barrel microswtich mount - front_v3 (Autodesk Fusion 360 design; units mm, degrees)
Autodesk Fusion 360 part; units mm, degrees
sketch "Sketch1" plane through (0, 0, 0) normal (0, 1, 0) x (1, 0, 0)
  line L0 (-4.4022, -9.8222) -> (-3.1214, -8.5414)
  arc A0 (10, -4.8314) -> (9.8222, -4.4022) centre (9.3929, -4.8314) ccw
  line L1 (6.5607, -5.5) -> (3.9, -2.8393)
  line L2 (-9.9987, -4.7917) -> (-10, -9.5)
  line L3 (9.8222, -4.4022) -> (8.5414, -3.1214)
  arc A1 (-3.2628, 8.2) -> (-3.1214, 8.5414) centre (-3.2628, 8.4) ccw
  line L4 (3.9, 2.8393) -> (6.5607, 5.5)
  arc A2 (-8.5414, 3.1214) -> (-8.2, 3.2628) centre (-8.4, 3.2628) ccw
  line L5 (-4.8314, 10) -> (-9.5, 10)
  line L6 (-6.5607, 5.5) -> (-3.9, 2.8393)
  arc A3 (-9.5, 10) -> (-10, 9.5) centre (-9.5, 9.5) ccw
  arc A4 (8.2, 3.2628) -> (8.5414, 3.1214) centre (8.4, 3.2628) ccw
  line L7 (-5.5, 6.5607) -> (-5.5, 8.2)
  line L8 (6.5607, 5.5) -> (8.2, 5.5)
  line L9 (8.5414, 3.1214) -> (9.8222, 4.4022)
  arc A5 (3.1214, 8.5414) -> (3.2628, 8.2) centre (3.2628, 8.4) ccw
  line L10 (-8.2, 3.2628) -> (-8.2, 5.5)
  line L11 (9.5, 10) -> (4.8314, 10)
  arc A6 (10, 9.5) -> (9.5, 10) centre (9.5, 9.5) ccw
  line L12 (10, 4.8314) -> (10, 9.5)
  arc A7 (-4.4312, 9.8494) -> (-4.8314, 10) centre (-4.8314, 9.3929) ccw
  line L13 (-9.8494, 4.4312) -> (-8.5414, 3.1214)
  line L14 (4.4022, 9.8222) -> (3.1214, 8.5414)
  line L15 (-5.5, 8.2) -> (-3.2628, 8.2)
  line L16 (5.5, 8.2) -> (5.5, 6.5607)
  arc A8 (-10, 4.9) -> (-9.8494, 4.4312) centre (-9.3734, 4.8428) ccw
  circle A9 centre (0, 0) radius 2.1
  arc A10 (4.8314, 10) -> (4.4022, 9.8222) centre (4.8314, 9.3929) ccw
  line L17 (-2.8393, 3.9) -> (-5.5, 6.5607)
  line L18 (5.5, 6.5607) -> (2.8393, 3.9)
  line L19 (-3.9, 2.8393) -> (-3.9, -2.8393)
  line L20 (-10, 9.5) -> (-10, 4.9)
  line L21 (2.8393, 3.9) -> (-2.8393, 3.9)
  line L22 (3.9, -2.8393) -> (3.9, 2.8393)
  line L23 (3.2628, 8.2) -> (5.5, 8.2)
  line L24 (8.2, 5.5) -> (8.2, 3.2628)
  line L25 (5.5, -6.5607) -> (5.5, -8.2)
  arc A11 (4.2336, -9.6536) -> (4.8314, -10) centre (4.8837, -9.2207) ccw
  arc A12 (-4.8314, -10) -> (-4.4022, -9.8222) centre (-4.8314, -9.3929) ccw
  line L26 (-5.5, -6.5607) -> (-2.8393, -3.9)
  line L27 (10, -9.5) -> (10, -4.8314)
  line L28 (-8.5414, -3.1214) -> (-9.8222, -4.4022)
  line L29 (5.5, -8.2) -> (3.2628, -8.2)
  line L30 (4.8314, -10) -> (9.5, -10)
  line L31 (-8.2, -5.5) -> (-8.2, -3.2628)
  arc A13 (8.5414, -3.1214) -> (8.2, -3.2628) centre (8.4, -3.2628) ccw
  line L32 (-2.8393, -3.9) -> (2.8393, -3.9)
  arc A14 (-8.2, -3.2628) -> (-8.5414, -3.1214) centre (-8.4, -3.2628) ccw
  arc A15 (-3.1214, -8.5414) -> (-3.2628, -8.2) centre (-3.2628, -8.4) ccw
  line L33 (3.1214, -8.5414) -> (4.2336, -9.6536)
  line L34 (-5.5, -8.2) -> (-5.5, -6.5607)
  line L35 (-6.5607, -5.5) -> (-8.2, -5.5)
  line L36 (8.2, -3.2628) -> (8.2, -5.5)
  arc A16 (-9.8222, -4.4022) -> (-9.9987, -4.7917) centre (-9.3929, -4.8314) ccw
  line L37 (-9.5, -10) -> (-4.8314, -10)
  arc A17 (-10, -9.5) -> (-9.5, -10) centre (-9.5, -9.5) ccw
  arc A18 (3.2628, -8.2) -> (3.1214, -8.5414) centre (3.2628, -8.4) ccw
  line L38 (8.2, -5.5) -> (6.5607, -5.5)
  line L39 (-3.2628, -8.2) -> (-5.5, -8.2)
  line L40 (-3.9, -2.8393) -> (-6.5607, -5.5)
  line L41 (2.8393, -3.9) -> (5.5, -6.5607)
  arc A19 (9.5, -10) -> (10, -9.5) centre (9.5, -9.5) ccw
  line L42 (-3.1214, 8.5414) -> (-4.4312, 9.8494)
  arc A20 (9.8222, 4.4022) -> (10, 4.8314) centre (9.3929, 4.8314) ccw
  line L43 (-8.2, 5.5) -> (-6.5607, 5.5)
  line L44 (4, 2.7979) -> (6.6021, 5.4)
  line L45 (6.6021, 5.4) -> (8.1, 5.4)
  line L46 (8.1, 5.4) -> (8.1, 3.2628)
  arc A21 (8.1, 3.2628) -> (8.6121, 3.0507) centre (8.4, 3.2628) ccw
  line L47 (8.6121, 3.0507) -> (9.8929, 4.3315)
  arc A22 (9.8929, 4.3315) -> (10.1, 4.8314) centre (9.3929, 4.8314) ccw
  line L48 (10.1, 4.8314) -> (10.1, 9.5)
  arc A23 (10.1, 9.5) -> (9.5, 10.1) centre (9.5, 9.5) ccw
  line L49 (9.5, 10.1) -> (4.8314, 10.1)
  arc A24 (4.8314, 10.1) -> (4.3315, 9.8929) centre (4.8314, 9.3929) ccw
  line L50 (4.3315, 9.8929) -> (3.0507, 8.6121)
  arc A25 (3.0507, 8.6121) -> (3.2628, 8.1) centre (3.2628, 8.4) ccw
  line L51 (3.2628, 8.1) -> (5.4, 8.1)
  line L52 (5.4, 8.1) -> (5.4, 6.6021)
  line L53 (5.4, 6.6021) -> (2.7979, 4)
  line L54 (2.7979, 4) -> (-2.7979, 4)
  line L55 (-2.7979, 4) -> (-5.4, 6.6021)
  line L56 (-5.4, 6.6021) -> (-5.4, 8.1)
  line L57 (-5.4, 8.1) -> (-3.2628, 8.1)
  arc A26 (-3.2628, 8.1) -> (-3.0509, 8.6124) centre (-3.2628, 8.4) ccw
  line L58 (-3.0509, 8.6124) -> (-4.3627, 9.9223)
  arc A27 (-4.3627, 9.9223) -> (-4.8314, 10.1) centre (-4.8314, 9.3929) ccw
  line L59 (-4.8314, 10.1) -> (-9.5, 10.1)
  arc A28 (-9.5, 10.1) -> (-10.1, 9.5) centre (-9.5, 9.5) ccw
  line L60 (-10.1, 9.5) -> (-10.1, 4.9044)
  arc A29 (-10.1, 4.9044) -> (-9.9226, 4.363) centre (-9.3734, 4.8428) ccw
  line L61 (-9.9226, 4.363) -> (-8.6124, 3.0509)
  arc A30 (-8.6124, 3.0509) -> (-8.1, 3.2628) centre (-8.4, 3.2628) ccw
  line L62 (-8.1, 3.2628) -> (-8.1, 5.4)
  line L63 (-8.1, 5.4) -> (-6.6021, 5.4)
  line L64 (-6.6021, 5.4) -> (-4, 2.7979)
  line L65 (-4, 2.7979) -> (-4, -2.7979)
  line L66 (-4, -2.7979) -> (-6.6021, -5.4)
  line L67 (-6.6021, -5.4) -> (-8.1, -5.4)
  line L68 (-8.1, -5.4) -> (-8.1, -3.2628)
  arc A31 (-8.1, -3.2628) -> (-8.6121, -3.0507) centre (-8.4, -3.2628) ccw
  line L69 (-8.6121, -3.0507) -> (-9.8929, -4.3315)
  arc A32 (-9.8929, -4.3315) -> (-10.0987, -4.7886) centre (-9.3929, -4.8314) ccw
  line L70 (-10.0987, -4.7886) -> (-10.1, -9.4997)
  arc A33 (-10.1, -9.4997) -> (-9.5, -10.1) centre (-9.5, -9.5) ccw
  line L71 (-9.5, -10.1) -> (-4.8314, -10.1)
  arc A34 (-4.8314, -10.1) -> (-4.3315, -9.8929) centre (-4.8314, -9.3929) ccw
  line L72 (-4.3315, -9.8929) -> (-3.0507, -8.6121)
  arc A35 (-3.0507, -8.6121) -> (-3.2628, -8.1) centre (-3.2628, -8.4) ccw
  line L73 (-3.2628, -8.1) -> (-5.4, -8.1)
  line L74 (-5.4, -8.1) -> (-5.4, -6.6021)
  line L75 (-5.4, -6.6021) -> (-2.7979, -4)
  line L76 (-2.7979, -4) -> (2.7979, -4)
  line L77 (2.7979, -4) -> (5.4, -6.6021)
  line L78 (5.4, -6.6021) -> (5.4, -8.1)
  line L79 (5.4, -8.1) -> (3.2628, -8.1)
  arc A36 (3.2628, -8.1) -> (3.0507, -8.6121) centre (3.2628, -8.4) ccw
  line L80 (3.0507, -8.6121) -> (4.1561, -9.7175)
  arc A37 (4.1561, -9.7175) -> (4.8282, -10.1) centre (4.8837, -9.2207) ccw
  line L81 (4.8282, -10.1) -> (9.5, -10.1)
  arc A38 (9.5, -10.1) -> (10.1, -9.5) centre (9.5, -9.5) ccw
  line L82 (10.1, -9.5) -> (10.1, -4.8314)
  arc A39 (10.1, -4.8314) -> (9.8929, -4.3315) centre (9.3929, -4.8314) ccw
  line L83 (9.8929, -4.3315) -> (8.6121, -3.0507)
  arc A40 (8.6121, -3.0507) -> (8.1, -3.2628) centre (8.4, -3.2628) ccw
  line L84 (8.1, -3.2628) -> (8.1, -5.4)
  line L85 (8.1, -5.4) -> (6.6021, -5.4)
  line L86 (6.6021, -5.4) -> (4, -2.7979)
  line L87 (4, -2.7979) -> (4, 2.7979)
  line L88 (9, 9) -> (25.1, 9)
  line L89 (25.1, 9) -> (25.1, -17)
  line L90 (25.1, -17) -> (9, -17)
  line L91 (9, -17) -> (9, 9)
  line L92 (10.1, -5.988) -> (10.1, -17)
  dimension "d1" = 0.1
  dimension "d2" = 16.1
  dimension "d3" = 26
  constraint horizontal L88
  constraint vertical L89
  constraint horizontal L90
  constraint vertical L91
  constraint coincident L82 L92.start
  constraint coincident L90 L92.end
  constraint perpendicular L90 L92
  measures "d2" distance of L88.start L88.end
  measures "d3" distance of L88.start L90.end
extrude "Extrude1" add sketch "Sketch1" along normal blind 25 contours L47 A22 L48 L82 A39 L83 L88 L89 L90 L91 L92 | L44 L45 L46 A21 L47 L83 A40 L84 L85 L86 L87 L91
fillet "Fillet1" radius 15 1 edges at (25.1, 12.5, -9)
sketch "Sketch2" plane through (0, 0, 17) normal (0, 0, 1) x (-1, 0, 0)
  line L0 (-10.1, 0) -> (-25.1, 0)
  line L1 (-25.1, 0) -> (-25.1, -25)
  line L2 (-25.1, -25) -> (-10.1, -25)
  line L3 (-10.1, -25) -> (-10.1, 0)
  line L4 (-10.1, 0) -> (-12.1, 0) construction
  line L5 (-12.1, 0) -> (-25.1, 0) construction
  line L6 (-18.6, 0) -> (-18.6, -25) construction
  line L7 (-25.1, -12.5) -> (-18.6, -12.5) construction
  line L8 (-25.1, -2.55) -> (-12.1, -2.55)
  line L9 (-12.1, -2.55) -> (-12.1, -22.45)
  line L10 (-12.1, -22.45) -> (-25.1, -22.45)
  line L11 (-25.1, -22.45) -> (-25.1, -2.55)
  line L12 (-25.1, -2.55) -> (-12.1, -22.45) construction
  line L13 (-12.1, -2.55) -> (-25.1, -22.45) construction
  line L14 (-12.1, -2.55) -> (-19.8, -2.55) construction
  line L15 (-19.8, -2.55) -> (-19.8, -22.45) construction
  line L16 (-19.8, -2.55) -> (-19.8, -7.7) construction
  line L17 (-19.8, -7.7) -> (-19.8, -17.3) construction
  line L18 (-19.8, -17.3) -> (-19.8, -22.45) construction
  circle A0 centre (-19.8, -7.7) radius 1.05
  circle A1 centre (-19.8, -17.3) radius 1.05
  line L19 (-12.1, -2.55) -> (-10.1, -2.55)
  line L20 (-10.1, -2.55) -> (-10.1, -22.45)
  line L21 (-10.1, -22.45) -> (-12.1, -22.45)
  line L22 (-12.1, -22.45) -> (-12.1, -2.55)
  point P0 (-18.6, -12.5)
  dimension "d8" = 2
  dimension "d9" = 19.9
  dimension "d10" = 7.7
  dimension "d11" = 5.15
  dimension "d12" = 9.6
  dimension "d13" = 5.15
  dimension "d14" = 2.1
  dimension "d15" = 2.1
  dimension "d16" = 19.9
  constraint coincident L0.start L3.end
  constraint perpendicular L3 L4
  constraint coincident L0.end L1.start
  constraint midpoint L5 L6.start
  constraint coincident L2 L6.end
  constraint perpendicular L2 L6
  constraint midpoint L1 L7.start
  constraint midpoint L6 P0
  constraint horizontal L8
  constraint perpendicular L8 L9
  constraint parallel L8 L10
  constraint parallel L9 L11
  constraint coincident L12 P0
  constraint coincident L13 P0
  constraint coincident P0 L7.end
  constraint perpendicular L9 L14
  constraint coincident L10 L15.end
  constraint perpendicular L10 L15
  constraint perpendicular L14 L16
  constraint perpendicular L7 L17
  constraint perpendicular L10 L18
  constraint coincident L16.end L17.start
  constraint coincident L17.end L18.start
  constraint horizontal L19
  constraint vertical L20
  constraint horizontal L21
  constraint vertical L22
  measures "d8" distance of L0.start L4.end
  measures "d9" distance of L8.end L9.end
  measures "d10" distance of L8.end L14.end
  measures "d11" distance of L14.end L16.end
  measures "d12" distance of L16.end L17.end
  measures "d13" distance of L17.end L15.end
  measures "d14" diameter of A0
  measures "d15" diameter of A1
  measures "d16" distance of L8.end L9.end
extrude "Extrude2" cut sketch "Sketch2" against normal blind 6.5 contours L3 L9 L19 L20 L21 L22 | L1 L8 L9 L10 L11 L22
sketch "Sketch3" plane through (0, 25, 0) normal (0, 1, 0) x (-1, 0, 0)
  arc A0 (-25.1, 6) -> (-10.1, -9) centre (-10.1, 6) ccw
  line L0 (-10.1, -9) -> (-10.1, -4.8314)
  arc A1 (-9.8929, -4.3315) -> (-10.1, -4.8314) centre (-9.3929, -4.8314) ccw
  line L1 (-9.8929, -4.3315) -> (-8.6121, -3.0507)
  arc A2 (-8.1, -3.2628) -> (-8.6121, -3.0507) centre (-8.4, -3.2628) ccw
  line L2 (-8.1, -3.2628) -> (-8.1, -5.4)
  line L3 (-8.1, -5.4) -> (-6.6021, -5.4)
  line L4 (-6.6021, -5.4) -> (-4, -2.7979)
  line L5 (-4, -2.7979) -> (-4, 2.7979)
  line L6 (-4, 2.7979) -> (-6.6021, 5.4)
  line L7 (-6.6021, 5.4) -> (-8.1, 5.4)
  line L8 (-8.1, 5.4) -> (-8.1, 3.2628)
  arc A3 (-8.6121, 3.0507) -> (-8.1, 3.2628) centre (-8.4, 3.2628) ccw
  line L9 (-8.6121, 3.0507) -> (-9.8929, 4.3315)
  arc A4 (-10.1, 4.8314) -> (-9.8929, 4.3315) centre (-9.3929, 4.8314) ccw
  line L10 (-10.1, 4.8314) -> (-10.1, 5.988)
  line L11 (-10.1, 5.988) -> (-10.1, 17)
  line L12 (-10.1, 17) -> (-25.1, 17)
  line L13 (-25.1, 17) -> (-25.1, 6)
  line L14 (-12.95, 2.8) -> (-11.05, 2.8)
  line L15 (-11.05, 2.8) -> (-11.05, -2.8)
  line L16 (-11.05, -2.8) -> (-12.95, -2.8)
  line L17 (-12.95, -2.8) -> (-12.95, 2.8)
  line L18 (-12.95, 2.8) -> (-11.05, -2.8) construction
  line L19 (-11.05, 2.8) -> (-12.95, -2.8) construction
  point P0 (-12, 0)
  dimension "d19" = 1.9
  dimension "d20" = 5.6
  constraint horizontal L14
  constraint perpendicular L14 L15
  constraint parallel L14 L16
  constraint parallel L15 L17
  constraint coincident L18 P0
  constraint coincident L19 P0
  measures "d19" distance of L15.end L16.end
  measures "d20" distance of L14.end L15.end
sketch "Sketch4" plane through (4, 0, 0) normal (-1, 0, 0) x (0, -1, 0)
  line L0 (0, -2.7979) -> (0, 2.7979)
  line L1 (0, 2.7979) -> (-25, 2.7979)
  line L2 (-25, 2.7979) -> (-25, -2.7979)
  line L3 (-25, -2.7979) -> (0, -2.7979)
  line L4 (0, 0) -> (-12.5, 0) construction
  circle A0 centre (-12.5, 0) radius 1.55
  circle A1 centre (-12.5, 0) radius 3
  dimension "d21" = 3.1
  dimension "d22" = 6
  constraint coincident L4.start origin
  constraint perpendicular L0 L4
  constraint coincident L4.end A0.centre
  measures "d21" diameter of A0
  measures "d22" diameter of A1
extrude "Extrude3" cut sketch "Sketch4" against normal blind 21 contours A0
extrude "Extrude4" cut sketch "Sketch4" against normal blind 10 from surface at -12 contours L3 A1 | L1 L3 A1 | L1 A1
extrude "Extrude5" cut sketch "Sketch3" against normal blind 15.5 contours L14 L15 L16 L17
